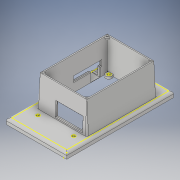
# Autodesk Inventor part: touchscreenCase
Saved by Autodesk Inventor 2019 (Build 230136000, 136)
## iProperties
Created: 2019-06-25
Part Number: touchscreenCase
Material: Generic
Document SubType Name: Modeling
Designer: Daniel
Density: 1 g/cm^3
Appearance: Default
Author: Daniel
Autodesk Inventor part; units mm, degrees
ref_plane "YZ Plane" through (0, 0, 0) normal (1, 0, 0) x (0, 1, 0)
sketch "Sketch1" plane through (0, 0, 0) normal (0, 1, 0) x (-1, 0, 0)
  line L0 (0, 0) -> (111.76, 0)
  line L1 (111.76, 0) -> (111.76, -198.12)
  line L2 (111.76, -198.12) -> (0, -198.12)
  line L3 (0, -198.12) -> (0, 0)
  dimension "d0" = 198.12
  dimension "d1" = 111.76
  constraints: 8 end point, 2 parallel, 1 horizontal, 1 perpendicular
  measures "d0" distance of L0.end L1.end
  measures "d1" distance of L0.start L0.end
extrude "Extrusion1" add sketch "Sketch1" along normal blind 10.668
shell "Shell1" thickness 2.54 removed faces 1 at (-37.2533, 0, -132.08)
ref_plane "Work Plane1" through (0, 67.818, 0) normal (0, 1, 0) x (1, 0, 0)
sketch "Sketch2" plane through (0, 67.818, 0) normal (0, 1, 0) x (1, 0, 0)
  line L0 (-111.76, 0) -> (0, 0) projected
  line L1 (0, 0) -> (0, 198.12) projected
  line L2 (0, 198.12) -> (-111.76, 198.12) projected
  line L3 (-111.76, 198.12) -> (-111.76, 0) projected
  line L4 (-111.76, 0) -> (-111.76, 198.12) construction
  line L5 (0, 198.12) -> (0, 0) construction
  line L6 (-111.76, 198.12) -> (0, 0) construction
  line L7 (0, 0) -> (-111.76, 0) construction
  line L8 (0, 0) -> (-111.76, 0) construction
  line L9 (-111.76, 0) -> (0, 198.12) construction
  line L10 (-111.76, 0) -> (0, 0) construction
  line L11 (0, 0) -> (0, 172.8125) construction
  line L12 (-111.76, 43.6372) -> (-111.76, 0) construction
  line L13 (0, 198.12) -> (-111.76, 198.12) construction
  line L14 (-111.76, 198.12) -> (-111.76, 175.26) construction
  line L15 (-95.7072, 173.99) -> (-9.525, 173.99) construction
  line L16 (0, 175.26) -> (0, 198.12) construction
  line L17 (-95.7072, 43.6372) -> (-9.525, 43.6372)
  line L18 (-98.8822, 170.815) -> (-98.8822, 46.8122)
  line L19 (-6.35, 170.815) -> (-6.35, 46.8122)
  arc A0 (-6.35, 170.815) -> (-9.525, 173.99) centre (-9.525, 170.815) ccw
  arc A1 (-95.7072, 173.99) -> (-98.8822, 170.815) centre (-95.7072, 170.815) ccw
  arc A2 (-98.8822, 46.8122) -> (-95.7072, 43.6372) centre (-95.7072, 46.8122) ccw
  arc A3 (-9.525, 43.6372) -> (-6.35, 46.8122) centre (-9.525, 46.8122) ccw
  line L20 (-9.525, 173.99) -> (-95.7072, 173.99)
  line L21 (-98.1482, 173.99) -> (-98.8822, 173.99)
  line L22 (-9.525, 170.815) -> (-95.7072, 170.815)
  line L23 (-95.7072, 170.815) -> (-95.7072, 46.8122)
  line L24 (-95.7072, 46.8122) -> (-9.525, 46.8122)
  line L25 (-9.525, 46.8122) -> (-9.525, 170.815)
  dimension "d7" = 24.13
  dimension "d28" = 43.6372
  dimension "d30" = 6.35
  dimension "d31" = 3.175
  constraints: 38 end point, 8 parallel, 8 point on circle, 8 tangent, 5 horizontal, 5 point on line, 4 centre point, 4 perpendicular, 3 equal radius, 1 collinear
  measures "d7" distance between parallel lines of L2 L15
  measures "d28" distance between parallel lines of L0 L17
  measures "d30" distance between parallel lines of L1 L19
  measures "d31" radius of A0
sketch "Sketch3" plane through (0, 10.668, 0) normal (0, 1, 0) x (1, 0, 0)
  circle A0 centre (-20.3962, 33.147) radius 1.905
  circle A1 centre (-20.3962, 164.7444) radius 1.905
  circle A2 centre (-86.7664, 33.147) radius 1.905
  circle A3 centre (-86.7664, 164.7444) radius 1.905
  line L0 (-111.76, 198.12) -> (-111.76, 0) projected
  line L1 (-111.76, 0) -> (0, 0) projected
  line L2 (0, 0) -> (0, 198.12) projected
  line L3 (0, 198.12) -> (-111.76, 198.12) projected
  circle A4 centre (-20.3962, 33.147) radius 3.175
  circle A5 centre (-86.7664, 33.147) radius 3.175
  circle A6 centre (-86.7664, 164.7444) radius 3.175
  circle A7 centre (-20.3962, 164.7444) radius 3.175
  dimension "d8" = 3.81
  dimension "d9" = 24.9936
  dimension "d10" = 33.147
  dimension "d11" = 20.3962
  dimension "d12" = 33.147
  dimension "d13" = 20.3962
  dimension "d14" = 33.3756
  dimension "d15" = 24.9936
  dimension "d16" = 33.3756
  dimension "d19" = 6.35
  constraints: 8 centre point, 6 equal radius, 4 coincident
  measures "d8" diameter of A1
  measures "d9" distance from line of L0 A2.centre
  measures "d10" distance from line of L1 A2.centre
  measures "d11" distance from line of L2 A0.centre
  measures "d12" distance from line of L1 A0.centre
  measures "d13" distance from line of L2 A1.centre
  measures "d14" distance from line of L3 A1.centre
  measures "d15" distance from line of L0 A3.centre
  measures "d16" distance from line of L3 A3.centre
  measures "d19" diameter of A7
extrude "Extrusion2" cut sketch "Sketch3" against normal blind 12.7 contours A0 | A1 | A2 | A3
sketch "Sketch4" plane through (0, 10.668, 0) normal (0, 1, 0) x (1, 0, 0)
  circle A0 centre (-20.3962, 33.147) radius 1.905 projected
  circle A1 centre (-86.7664, 164.7444) radius 1.905 projected
  circle A2 centre (-20.3962, 33.147) radius 1.905 projected
  circle A3 centre (-86.7664, 33.147) radius 1.905 projected
  circle A4 centre (-20.3962, 164.7444) radius 1.905 projected
  line L0 (-111.76, 0) -> (0, 0) projected
  line L1 (0, 0) -> (0, 198.12) projected
  line L2 (0, 198.12) -> (-111.76, 198.12) projected
  line L3 (-111.76, 198.12) -> (-111.76, 0) projected
  circle A5 centre (-20.3962, 33.147) radius 3.175
  circle A6 centre (-86.7664, 33.147) radius 3.175
  circle A7 centre (-86.7664, 164.7444) radius 3.175
  circle A8 centre (-20.3962, 164.7444) radius 3.175
  dimension "d20" = 6.35
  constraints: 4 centre point, 4 coincident, 3 equal radius
  measures "d20" diameter of A8
extrude "Extrusion3" cut sketch "Sketch4" against normal blind 2.032 contours A5 | A6 | A7 | A8
move faces "Move1" translate (0, -1.27, 0) faces at (-42.7448, 8.128, -77.6065)
fillet "Fillet1" radius 4.7625 4 edges at (-55.88, 10.668, 0) (-111.76, 10.668, -99.06) (0, 10.668, -99.06) (-55.88, 10.668, -198.12)
sketch "Sketch6" plane through (0, 10.668, 0) normal (0, 1, 0) x (1, 0, 0)
  circle A0 centre (-20.3962, 164.7444) radius 3.175 projected
  circle A1 centre (-86.7664, 33.147) radius 3.175 projected
  circle A2 centre (-20.3962, 33.147) radius 3.175 projected
  circle A3 centre (-86.7664, 164.7444) radius 3.175 projected
  line L0 (-106.9975, 193.3575) -> (-4.7625, 193.3575) projected
  line L1 (-106.9975, 4.7625) -> (-106.9975, 193.3575) projected
  line L2 (-4.7625, 4.7625) -> (-106.9975, 4.7625) projected
  line L3 (-4.7625, 193.3575) -> (-4.7625, 4.7625) projected
  point P0 (0, 0)
extrude "Extrusion4" add sketch "Sketch2" against normal blind 57.15 contours A2 L18 A1 L20 A0 L19 A3 L17
offset faces "Size1" outward 1.905 faces at (-9.525, 48.768, -88.1465) (-38.2524, 48.768, -170.815) (-66.9798, 48.768, -46.8122) (-95.7072, 48.768, -129.4807)
draft "FaceDraft1" angle 3 pull direction (0, 1, 0) faces at (-66.9798, 48.768, -173.99) (-6.3589, 29.718, -171.0523) (-98.0346, 29.718, -172.9745) (-6.35, 29.718, -129.4807) (-98.8822, 29.718, -88.1465) (-6.3589, 48.768, -46.5749) (-97.4957, 29.718, -44.1889) (-38.2524, 48.768, -43.6372) fixed edges at (-52.6161, 10.668, -173.99) (-7.2799, 10.668, -173.0601) (-97.9523, 10.668, -173.0601) (-6.35, 10.668, -108.8136) (-98.8822, 10.668, -108.8136) (-7.2799, 10.668, -44.5671) (-97.9523, 10.668, -44.5671) (-52.6161, 10.668, -43.6372)
sketch "Sketch7" plane through (-95.7072, 67.818, -46.6323) normal (0, 0.052336, 0.9986295) x (1, 0, 0)
  line L0 (31.6484, -53.647) -> (79.9084, -53.647)
  line L1 (79.9084, -53.647) -> (79.9084, -29.7456)
  line L2 (79.9084, -29.7456) -> (31.6484, -29.7456)
  line L3 (31.6484, -29.7456) -> (31.6484, -53.647)
  line L4 (86.1822, -57.2284) -> (0, -57.2284) projected
  line L5 (86.1822, 0) -> (86.1822, -57.2284) projected
  point P0 (95.7072, -70.1656)
  dimension "d36" = 3.5814
  dimension "d37" = 23.9014
  dimension "d38" = 48.26
  dimension "d39" = 6.2738
  constraints: 8 end point, 2 parallel, 1 horizontal, 1 perpendicular
  measures "d36" distance between parallel lines of L4 L0
  measures "d37" distance between parallel lines of L0 L2
  measures "d38" distance between parallel lines of L1 L3
  measures "d39" distance between parallel lines of L5 L1
extrude "Extrusion5" cut sketch "Sketch7" against normal blind 7.9375
chamfer "Chamfer1" distance 1.27 angle 45 8 edges at (-15.7988, 26.1788, -44.4501) (-39.9288, 38.1131, -45.0755) (-39.9288, 14.2445, -43.8246) (-39.9288, 13.9881, -48.7172) (-64.0588, 26.1788, -44.4501) (-64.0588, 25.9552, -48.7172) (-15.7988, 25.9552, -48.7172) (-39.9288, 37.9223, -48.7172)
sketch "Sketch8" plane through (-95.8871, 67.818, -170.815) normal (-0.9986295, 0.052336, 0) x (0, 0, 1)
  line L0 (12.8524, -34.9032) -> (63.6524, -34.9032)
  line L1 (63.6524, -34.9032) -> (63.6524, -43.6662)
  line L2 (12.8524, -43.6662) -> (12.8524, -34.9032)
  line L3 (33.3461, -34.9032) -> (44.7303, -34.9032)
  line L4 (31.7754, -43.6662) -> (31.7754, -60.3032)
  line L5 (31.7754, -60.3032) -> (15.9004, -60.3032)
  line L6 (15.9004, -60.3032) -> (15.9004, -43.6662)
  line L7 (63.6524, -43.6662) -> (31.7754, -43.6662)
  line L8 (15.9004, -43.6662) -> (12.8524, -43.6662)
  line L9 (0, 0) -> (0, -57.2284) projected
  point P0 (170.815, -62.7067)
  dimension "d49" = 15.875
  dimension "d50" = 50.8
  dimension "d51" = 25.4
  dimension "d53" = 3.048
  dimension "d54" = 8.763
  dimension "d55" = 12.8524
  constraints: 18 end point, 5 parallel, 2 horizontal, 2 perpendicular, 1 collinear, 1 point on line
  measures "d49" distance between parallel lines of L4 L6
  measures "d50" distance between parallel lines of L1 L2
  measures "d51" distance between parallel lines of L0 L5
  measures "d53" distance between parallel lines of L6 L2
  measures "d54" distance between parallel lines of L7 L0
  measures "d55" distance between parallel lines of L9 L2
extrude "Extrusion6" cut sketch "Sketch8" along normal blind 30.1625 and the other way blind 19.3421
sketch "Sketch9" plane through (0, 10.668, 0) normal (0, 1, 0) x (1, 0, 0)
  line L0 (-93.8022, 168.91) -> (-93.8022, 154.9146) projected
  line L1 (-93.8022, 48.7172) -> (-11.43, 48.7172) projected
  line L2 (-11.43, 48.7172) -> (-11.43, 168.91) projected
  line L3 (-11.43, 168.91) -> (-93.8022, 168.91) projected
  circle A0 centre (-20.3962, 164.7444) radius 3.175 projected
  circle A1 centre (-86.7664, 164.7444) radius 3.175 projected
  line L4 (-11.43, 168.91) -> (-93.8022, 168.91) projected
  line L5 (-11.43, 168.91) -> (-11.43, 48.7172) projected
  line L6 (-24.1122, 168.91) -> (-82.7168, 168.91)
  arc A2 (-24.0722, 168.9453) -> (-15.3337, 167.0964) centre (-20.3962, 164.7444) ccw
  arc A3 (-91.7655, 167.7042) -> (-82.7168, 168.91) centre (-86.7664, 164.7444) ccw
  line L7 (-11.43, 48.7172) -> (-11.43, 168.91) projected
  line L8 (-11.43, 48.7172) -> (-93.8022, 48.7172)
  line L9 (-93.8022, 168.91) -> (-93.8022, 48.7172) projected
  line L10 (-93.8022, 48.7172) -> (-93.8022, 168.91)
  line L11 (-11.43, 168.91) -> (-15.3337, 167.0964)
  line L12 (-93.8022, 168.91) -> (-91.7655, 167.7042)
  line L13 (-79.5136, 139.0396) -> (-93.8022, 139.0396) projected
  line L14 (-93.8022, 139.0396) -> (-93.8022, 48.7172) projected
  line L15 (-93.8022, 154.9146) -> (-79.5136, 154.9146) projected
  line L16 (-79.5136, 154.9146) -> (-79.5136, 139.0396) projected
  point P0 (0, 0)
  constraints: 10 end point, 5 point on circle, 2 centre point, 2 coincident, 2 collinear, 1 perpendicular
extrude "Extrusion7" cut sketch "Sketch9" against normal blind 30.1625 contours L12 A3 L3 A2 L11 L2 L1 L9 L13 L16 L15 L0 | L15 L16 L13 L9
fillet "Fillet2" radius 1.905 4 edges at (-109.22, 0, -99.06) (-55.88, 0, -195.58) (-2.54, 0, -99.06) (-55.88, 0, -2.54)
ref_plane "Work Plane2" through (0, 0, -198.12) normal (-1, 0, 0) x (0, 0, 1)
chamfer "Chamfer3" distance 1.016 angle 45 14 edges at (-93.8022, 15.6527, -154.9146) (-98.5273, 17.4398, -154.9146) (-97.9431, 28.5872, -157.9626) (-93.8022, 28.3702, -157.9626) (-98.5273, 17.4398, -139.0396) (-98.1724, 24.2117, -123.1011) (-93.8022, 23.9826, -123.1011) (-93.8022, 15.6527, -139.0396) (-97.9431, 28.5872, -107.1626) (-93.8022, 28.3702, -107.1626) (-93.8022, 32.7577, -132.5626) (-97.7138, 32.9627, -132.5626) (-95.9873, 24.0972, -154.9146) (-95.9873, 24.0972, -139.0396)
fillet "Fillet3" radius 1.905 6 edges at (-109.4059, 10.0141, -154.9146) (-102.9399, 10.668, -154.9146) (-98.3735, 10.668, -154.9146) (-109.4059, 10.0141, -139.0396) (-102.9399, 10.668, -139.0396) (-98.3735, 10.668, -139.0396)
chamfer "Chamfer4" distance 1.016 angle 45 2 edges at (-98.1724, 24.2117, -157.4546) (-93.8022, 23.9826, -157.4546)
fillet "Fillet4" radius 1.905 1 edges at (-111.153, 8.2321, -146.9771)
sketch "Sketch13" plane through (0, 67.818, 0) normal (0, 1, 0) x (1, 0, 0)
  arc A0 (-9.3451, 170.815) -> (-9.525, 170.9949) centre (-9.525, 170.815) ccw construction
  arc A1 (-95.7072, 170.9949) -> (-95.8871, 170.815) centre (-95.7072, 170.815) ccw construction
  line L0 (-9.525, 170.815) -> (-95.7072, 170.815) construction
  arc A2 (-95.8871, 46.8122) -> (-95.7072, 46.6323) centre (-95.7072, 46.8122) ccw construction
  line L1 (-95.7072, 170.815) -> (-95.7072, 46.8122) construction
  arc A3 (-9.525, 46.6323) -> (-9.3451, 46.8122) centre (-9.525, 46.8122) ccw construction
  line L2 (-95.7072, 46.8122) -> (-9.525, 46.8122) construction
  line L3 (-9.525, 46.8122) -> (-9.525, 170.815) construction
  line L4 (-9.525, 170.815) -> (-95.7072, 46.8122) construction
  line L5 (-95.7072, 170.815) -> (-9.525, 46.8122) construction
  arc A4 (-15.875, 170.815) -> (-9.525, 164.465) centre (-9.525, 170.815) ccw
  arc A5 (-95.7072, 164.465) -> (-89.3572, 170.815) centre (-95.7072, 170.815) ccw
  arc A6 (-89.3572, 46.8122) -> (-95.7072, 53.1622) centre (-95.7072, 46.8122) ccw
  arc A7 (-9.525, 53.1622) -> (-15.875, 46.8122) centre (-9.525, 46.8122) ccw
  line L6 (-89.3572, 170.815) -> (-95.7072, 170.815)
  line L7 (-95.7072, 164.465) -> (-95.7072, 170.815)
  line L8 (-9.525, 170.815) -> (-15.875, 170.815)
  line L9 (-9.525, 164.465) -> (-9.525, 170.815)
  line L10 (-9.525, 53.1622) -> (-9.525, 46.8122)
  line L11 (-9.525, 46.8122) -> (-15.875, 46.8122)
  line L12 (-95.7072, 53.1622) -> (-95.7072, 46.8122)
  line L13 (-95.7072, 46.8122) -> (-89.3572, 46.8122)
  point P0 (0, 0)
  dimension "d80" = 6.35
  dimension "d81" = 6.35
  dimension "d82" = 6.35
  dimension "d83" = 6.35
  constraints: 28 end point, 8 point on circle, 8 point on line, 5 perpendicular, 4 centre point, 4 coincident, 4 collinear, 1 horizontal, 1 vertical
  measures "d80" radius of A4
  measures "d81" radius of A5
  measures "d82" radius of A6
  measures "d83" radius of A7
extrude "Extrusion9" add sketch "Sketch13" against normal blind 6.35
fillet "Fillet5" radius 3.175 4 edges at (-91.2171, 61.468, -166.3249) (-14.0151, 61.468, -166.3249) (-14.0151, 61.468, -51.3023) (-91.2171, 61.468, -51.3023)
sketch "Sketch14" plane through (0, 67.818, 0) normal (0, 1, 0) x (1, 0, 0)
  circle A0 centre (-12.1326, 168.2166) radius 1.905
  circle A1 centre (-93.0773, 168.2166) radius 1.905
  circle A2 centre (-93.0773, 49.4421) radius 1.905
  circle A3 centre (-12.1326, 49.4198) radius 1.905
  line L0 (-15.5556, 168.91) -> (-11.43, 164.7955) construction
  line L1 (-89.6497, 168.91) -> (-93.8022, 164.7955) construction
  line L2 (-93.8022, 52.8697) -> (-89.6497, 48.7172) construction
  arc A4 (-11.43, 52.8697) -> (-15.5825, 48.7172) centre (-9.525, 46.8122) ccw construction
  line L3 (-11.43, 52.8697) -> (-15.5825, 48.7172) construction
  point P0 (0, 0)
  dimension "d87" = 3.81
  constraints: 8 end point, 4 centre point, 3 equal radius
  measures "d87" diameter of A3
extrude "Extrusion10" cut sketch "Sketch14" against normal blind 4.445
sketch "Sketch15" plane through (-9.3451, 67.818, -46.8122) normal (0.9986295, 0.052336, 0) x (0, 0, -1)
  point P0 (-46.8122, -68.2141)
body "Solid1"
